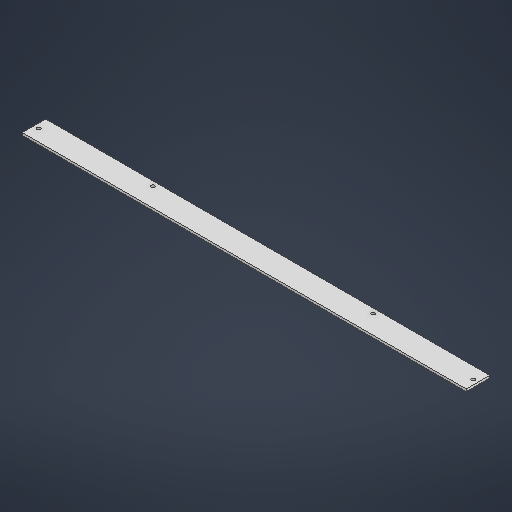
# Autodesk Inventor part: PCB_Kabelkanaldeckel_1.0
Saved by Autodesk Inventor 2027 (Build 310192060, 192F)
## iProperties
Created: 2026-05-05
Part Number: PCB_Kabelkanaldeckel_1.0
Material: Generisch
Document SubType Name: Modeling
Designer: simon
Density: 1 g/cm^3
Appearance: Vorgabe
Author: simon
Autodesk Inventor part; units mm, degrees
ref_plane "YZ Plane" through (0, 0, 0) normal (1, 0, 0) x (0, 1, 0)
ref_plane "XZ Plane" through (0, 0, 0) normal (0, 1, 0) x (-1, 0, 0)
ref_plane "XY Plane" through (0, 0, 0) normal (0, 0, 1) x (1, 0, 0)
sketch "Skizze1" plane through (0, 0, 0) normal (0, 0, 1) x (1, 0, 0)
  line L0 (-188.78, 10) -> (188.78, 10)
  line L1 (188.78, 10) -> (188.78, -10)
  line L2 (188.78, -10) -> (-188.78, -10)
  line L3 (-188.78, -10) -> (-188.78, 10)
  line L4 (0, -14) -> (0, 14) construction
  line L5 (-264.292, 0) -> (264.292, 0) construction
  point P0 (0, 0)
  dimension "d0" = 377.56
  dimension "d1" = 20
  constraints: 8 end point, 2 parallel, 1 horizontal, 1 perpendicular, 2 other
  measures "d0" distance between parallel lines of L1 L3
  measures "d1" distance of L2.end L0.start
extrude "Extrusion1" add sketch "Skizze1" along normal blind 2
sketch "Skizze3" plane through (0, 0, 2) normal (0, 0, 1) x (1, 0, 0)
  circle A0 centre (-184.78, 0) radius 1.5
  line L0 (-188.78, 10) -> (-188.78, -10) projected
  line L1 (-264.292, 0) -> (264.292, 0) projected
  circle A1 centre (-93.64, 6) radius 1.5
  line L2 (188.78, 10) -> (-188.78, 10) projected
  line L3 (0, -14) -> (0, 14) projected
  point P0 (0, 0)
  dimension "d8" = 3
  dimension "d9" = 4
  dimension "d10" = 3
  dimension "d11" = 4
  dimension "d12" = 95.14
  dimension "d13" = 93.64
  constraints: 2 centre point, 1 point on line
  measures "d8" diameter of A0
  measures "d9" distance from line of L0 A0.centre
  measures "d10" diameter of A1
  measures "d11" distance from line of L2 A1.centre
  measures "d12" distance from line of L0 A1.centre
  measures "d13" distance from line of L3 A1.centre
extrude "Extrusion3" cut sketch "Skizze3" against normal through all contours L1 A0 | A0 L1 | A1
mirror "Spiegeln2" about plane through (0, 0, 0) normal (1, 0, 0) of "Extrusion3"
sketch "Skizze4" plane through (0, 0, 0) normal (0, 0, -1) x (-1, 0, 0)
  line L0 (187.28, 8.2503) -> (187.28, 3.5)
  line L1 (187.28, 3.5) -> (185.78, 3.5)
  line L2 (185.78, 3.5) -> (185.78, 7)
  line L3 (185.78, 7) -> (182.28, 7)
  line L4 (182.28, 7) -> (182.28, 8.5)
  line L5 (182.28, 8.5) -> (187.28, 8.5)
  line L6 (187.28, 8.5) -> (187.28, 8.2503)
  line L7 (188.78, 10) -> (188.78, -10) projected
  line L8 (-188.78, 10) -> (188.78, 10) projected
  point P0 (0, 0)
  dimension "d16" = 1.5
  dimension "d17" = 1.5
  dimension "d18" = 1.5
  dimension "d19" = 1.5
  dimension "d20" = 5
  dimension "d21" = 5
  constraints: 14 end point, 5 perpendicular, 1 collinear, 1 point on line, 1 vertical
  measures "d16" distance between parallel lines of L7 L0
  measures "d17" distance between parallel lines of L8 L5
  measures "d18" distance between parallel lines of L3 L5
  measures "d19" distance between parallel lines of L0 L2
  measures "d20" distance between parallel lines of L5 L1
  measures "d21" distance between parallel lines of L0 L4
extrude "Extrusion4" add sketch "Skizze4" along normal blind 1
mirror "Spiegeln3" about plane through (0, 0, 0) normal (1, 0, 0) of "Extrusion4"
mirror "Spiegeln5" about plane through (0, 0, 0) normal (0, 1, 0) of "Extrusion4", "Spiegeln3"
sketch "Skizze5" plane through (-182.28, -8.5, -1) normal (0, 0, -1) x (-1, 0, 0)
  line L0 (0, 1.5) -> (3.5, 1.5) projected
  line L1 (5, 0) -> (0, 0) projected
  line L2 (3.5, 1.5) -> (0, 1.5)
  line L3 (0, 1.5) -> (0, 0)
  line L4 (0, 0) -> (3.5, 0)
  line L5 (3.5, 0) -> (3.5, 1.5)
  point P0 (-182.28, 8.5)
  constraints: 8 end point, 2 parallel, 1 horizontal, 1 perpendicular
extrude "Extrusion5" cut sketch "Skizze5" against normal blind 1
